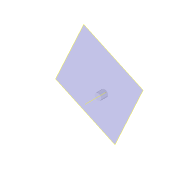
# Autodesk Inventor part: 00_KES400_Lens
Saved by Autodesk Inventor 2022 (Build 260153000, 153)
## iProperties
Created: 2019-04-29
Part Number: 00_KES400_Lens
Material: Generic
Document SubType Name: Modeling
Designer: diederichbenedict
Density: 1 g/cm^3
Appearance: Polycarbonate - Clear
Author: diederichbenedict
Autodesk Inventor part; units mm, degrees
ref_plane "YZ Plane" through (0, 0, 0) normal (1, 0, 0) x (0, 1, 0)
ref_plane "XZ Plane" through (0, 0, 0) normal (0, 1, 0) x (-1, 0, 0)
ref_plane "XY Plane" through (0, 0, 0) normal (0, 0, 1) x (1, 0, 0)
ref_plane "Work Plane1" through (15.8127, -3.2465, 0) normal (0, 0, -1) x (0.417504, 0.9086751, 0)
sketch "Sketch1" plane through (15.8127, -3.2465, 0) normal (0, 0, -1) x (0.417504, 0.9086751, 0)
  line L0 (-7.897, -2) -> (1.603, -2) projected
  line L1 (1.603, -2) -> (1.603, -5.5) projected
  line L2 (1.603, -5.5) -> (-7.897, -5.5) projected
  line L3 (-7.897, -5.5) -> (-7.897, -2) projected
  line L4 (1.603, -19) -> (-7.897, -19) projected
  line L5 (-7.897, -19) -> (-7.897, -15.5) projected
  line L6 (-7.897, -15.5) -> (1.603, -15.5) projected
  line L7 (1.603, -15.5) -> (1.603, -19) projected
  arc A0 (9.303, -26.8555) -> (8.303, -25.8555) centre (8.303, -26.8555) ccw projected
  line L8 (9.303, -26.8555) -> (9.303, -30) projected
  line L9 (9.303, -30) -> (-16.397, -30) projected
  line L10 (-16.397, -30) -> (-16.397, -20.4723) projected
  arc A1 (-15.397, -19.4723) -> (-16.397, -20.4723) centre (-15.397, -20.4723) ccw projected
  line L11 (-15.397, -19.4723) -> (-13.5347, -19.4723) projected
  arc A2 (-13.5347, -19.4723) -> (-12.5347, -18.4723) centre (-13.5347, -18.4723) ccw projected
  line L12 (-12.5347, -18.4723) -> (-12.5347, 0) projected
  line L13 (-12.5347, 0) -> (-1, 0) projected
  arc A3 (-1, 0) -> (0, 1) centre (-1, 1) ccw projected
  line L14 (0, 1) -> (0, 2) projected
  arc A4 (1, 3) -> (0, 2) centre (1, 2) ccw projected
  line L15 (1, 3) -> (3.5653, 3) projected
  arc A5 (4.5653, 2) -> (3.5653, 3) centre (3.5653, 2) ccw projected
  line L16 (4.5653, 2) -> (4.5653, -24.8555) projected
  arc A6 (4.5653, -24.8555) -> (5.5653, -25.8555) centre (5.5653, -24.8555) ccw projected
  line L17 (5.5653, -25.8555) -> (8.303, -25.8555) projected
  line L18 (2.603, -17.5) -> (2.603, -2) projected
  line L19 (2.603, -2) -> (-10.897, -2) projected
  line L20 (-10.897, -2) -> (-10.897, -17.5) projected
  line L21 (-10.897, -17.5) -> (2.603, -17.5) projected
  circle A7 centre (6.603, -27.5) radius 1 projected
  circle A8 centre (-13.897, -21) radius 1 projected
  circle A9 centre (1.603, 0.5) radius 1 projected
  circle A10 centre (-3.397, -10) radius 2.6486
  point P0 (-3.6519, -15.7241)
  dimension "d0" = 10.5
  dimension "d1" = 11
  dimension "d2" = 10.5
  dimension "d3" = 5
  constraints: 1 centre point
  measures "d0" vertical distance of A10.centre A9.centre
  measures "d1" vertical distance of A8.centre A10.centre
  measures "d2" horizontal distance of A8.centre A10.centre
  measures "d3" horizontal distance of A10.centre A9.centre
extrude "Extrusion1" add sketch "Sketch1" against normal up to surface (5.5 mm away) contours A10
body "Solid1"
